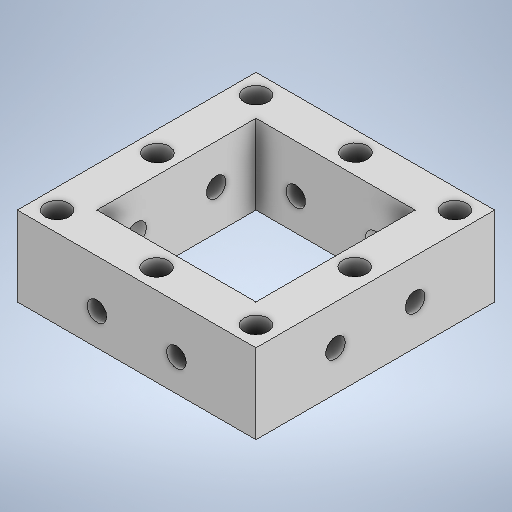
# Autodesk Inventor part: sleeve
Saved by Autodesk Inventor 2025.2 (Build 292293000, 293)
## iProperties
Created: 2026-03-22
Part Number: sleeve
Material: Generic
Document SubType Name: Modeling
Designer: hp
Density: 1 g/cm^3
Appearance: Default
Author: hp
Autodesk Inventor part; units mm, degrees
ref_plane "YZ Plane" through (0, 0, 0) normal (1, 0, 0) x (0, 1, 0)
ref_plane "XZ Plane" through (0, 0, 0) normal (0, 1, 0) x (-1, 0, 0)
ref_plane "XY Plane" through (0, 0, 0) normal (0, 0, 1) x (1, 0, 0)
sketch "Sketch1" plane through (0, 0, 0) normal (0, 1, 0) x (-1, 0, 0)
  line L0 (10, -10) -> (-10, -10)
  line L1 (-10, -10) -> (-10, 10)
  line L2 (-10, 10) -> (10, 10)
  line L3 (10, 10) -> (10, -10)
  line L4 (10, -10) -> (-10, 10) construction
  line L5 (-10, -10) -> (10, 10) construction
  line L6 (-15, 15) -> (15, 15)
  line L7 (15, 15) -> (15, -15)
  line L8 (15, -15) -> (-15, -15)
  line L9 (-15, -15) -> (-15, 15)
  line L10 (-15, 15) -> (15, -15) construction
  line L11 (15, 15) -> (-15, -15) construction
  circle A0 centre (12.4, 0) radius 1.5
  circle A1 centre (0, 12.5) radius 1.5
  circle A2 centre (0, -12.5) radius 1.5
  circle A3 centre (12.5, -12.5) radius 1.5
  circle A4 centre (12.5, 12.5) radius 1.5
  line L12 (0, -15) -> (0, 15)
  circle A5 centre (-12.4, 0) radius 1.5
  circle A6 centre (-12.5, -12.5) radius 1.5
  circle A7 centre (-12.5, 12.5) radius 1.5
  point P0 (0, 0)
  point P1 (10, 0)
  dimension "d0" = 20
  dimension "d1" = 20
  dimension "d4" = 30
  dimension "d5" = 30
  dimension "d6" = 3
  dimension "d7" = 3
  dimension "d8" = 3
  dimension "d9" = 12.5
  dimension "d10" = 12.4
  dimension "d11" = 12.5
  dimension "d12" = 3
  dimension "d13" = 3
  dimension "d14" = 12.5
  constraints: 26 end point, 8 centre point, 7 midpoint, 4 parallel, 3 symmetric about line, 2 horizontal, 2 perpendicular, 2 point on line, 3 other
  measures "d0" distance of L1.end L2.end
  measures "d1" distance of L0.end L1.end
  measures "d4" distance of L7.end L8.end
  measures "d5" distance of L6.end L7.end
  measures "d6" diameter of A0
  measures "d7" diameter of A1
  measures "d8" diameter of A2
  measures "d9" distance of point (0, 0) A2.centre
  measures "d10" distance of point (0, 0) A0.centre
  measures "d11" distance of point (0, 0) A1.centre
  measures "d12" diameter of A3
  measures "d13" diameter of A4
  measures "d14" horizontal distance of point (0, 0) A4.centre
extrude "Extrusion1" add sketch "Sketch1" along normal mid plane 10 contours L3 L2 L12 A1 L6 L7 L8 A2 L0 | L12 A2 L8 L9 L6 A1 L2 L1 L0
sketch "Sketch2" plane through (-15, 5, 15) normal (0, 0, 1) x (1, 0, 0)
  line L0 (30, 0) -> (30, -10) projected
  line L1 (0, 0) -> (30, 0) projected
  line L2 (0, -10) -> (0, 0) projected
  line L3 (30, -10) -> (0, -10) projected
  point P0 (15, -5)
  point P1 (10, -6)
  point P2 (20, -6)
  dimension "d17" = 10
  dimension "d18" = 10
  measures "d17" distance from line of point (10, -6) L2
  measures "d18" distance from line of L0 point (20, -6)
hole "Hole1" at (5, -1, 15) at (-5, -1, 15) direction (0, 0, -1) diameter 2.45 depth 30
sketch "Sketch3" plane through (15, -5, -15) normal (1, 0, 0) x (0, 0, -1)
  line L0 (0, 0) -> (0, 10) projected
  point P0 (-15, 5)
  point P1 (-20, 5)
  point P2 (-10, 5)
  point P3 (0, 5)
  dimension "d26" = 10
  dimension "d27" = 10
  constraints: 1 midpoint
  measures "d26" distance of point (0, 5) point (-10, 5)
  measures "d27" distance of point (-10, 5) point (-20, 5)
hole "Hole2" at (15, 0, -5) at (15, 0, 5) direction (-1, 0, 0) diameter 2.45 depth 30
body "Solid1"
